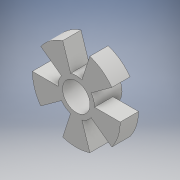
# Autodesk Inventor part: Encoder_helice
Saved by Autodesk Inventor 2017 (Build 210142000, 142)
## iProperties
Created: 2016-07-30
Part Number: Encoder_helice
Material: Generic
Document SubType Name: Modeling
Designer: ANDRES
Density: 1 g/cm^3
Appearance: Default
Author: ANDRES
Autodesk Inventor part; units mm, degrees
ref_plane "YZ Plane" through (0, 0, 0) normal (1, 0, 0) x (0, 1, 0)
ref_plane "XZ Plane" through (0, 0, 0) normal (0, 1, 0) x (-1, 0, 0)
ref_plane "XY Plane" through (0, 0, 0) normal (0, 0, 1) x (1, 0, 0)
sketch "Sketch2" plane through (0, 0, 0) normal (0, 1, 0) x (-1, 0, 0)
  circle A0 centre (0, 0) radius 4.8
  line L0 (1.618, 1.1756) -> (3.8833, 2.8214)
  line L1 (0.618, 1.9021) -> (1.4833, 4.5651)
  line L2 (-0.618, 1.9021) -> (-1.4833, 4.5651)
  line L3 (-1.618, 1.1756) -> (-3.8833, 2.8214)
  line L4 (-2, 0) -> (-4.8, 0)
  line L5 (1.618, -1.1756) -> (3.8833, -2.8214)
  line L6 (0.618, -1.9021) -> (1.4833, -4.5651)
  line L7 (-0.618, -1.9021) -> (-1.4833, -4.5651)
  line L8 (-1.618, -1.1756) -> (-3.8833, -2.8214)
  arc A1 (2, 0) -> (1.618, 1.1756) centre (0, 0) ccw
  arc A2 (0.618, -1.9021) -> (1.618, -1.1756) centre (0, 0) ccw
  arc A3 (-1.618, -1.1756) -> (-0.618, -1.9021) centre (0, 0) ccw
  arc A4 (0.618, 1.9021) -> (-0.618, 1.9021) centre (0, 0) ccw
  arc A5 (-1.618, 1.1756) -> (-2, 0) centre (0, 0) ccw
  line L9 (2, 0) -> (4.8, 0)
  dimension "d22" = 9.6
  constraints: 20 end point, 10 point on circle, 5 centre point, 3 coincident, 1 horizontal, 12 other
extrude "Extrusion1" add sketch "Sketch2" along normal blind 2 contours A0 L5 A2 L6 L7 A3 L8 L4 A5 L3 L2 A4 L1 L0 A1 L9
sketch "Sketch3" plane through (0, 2, 0) normal (0, 1, 0) x (1, 0, 0)
  circle A0 centre (0, 0) radius 2
  circle A1 centre (0, 0) radius 1.5
  dimension "d39" = 3
  dimension "d44" = 4
  constraints: 2 centre point, 2 coincident
  measures "d39" diameter of A1
  measures "d44" diameter of A0
extrude "Extrusion2" add sketch "Sketch3" along normal blind 1 contours A0 | A1
extrude "Extrusion3" cut sketch "Sketch3" along normal blind 1 and the other way blind 2 contours A1
body "Solid1"
